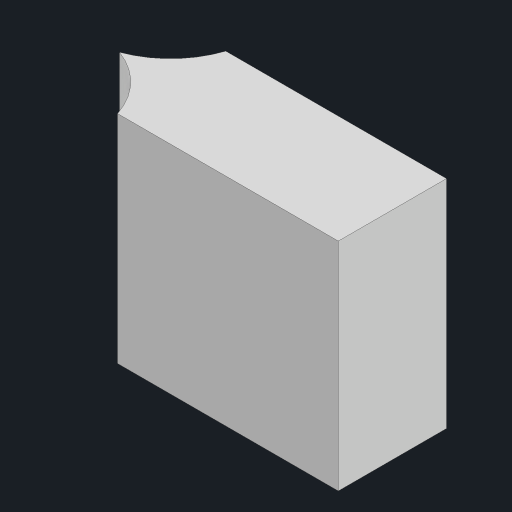
# Autodesk Inventor part: Capper Gate
Saved by Autodesk Inventor 2023.1 (Build 271208000, 208)
## iProperties
Created: 2023-02-21
Part Number: Capper Gate
Material: Generic
Document SubType Name: Modeling
Designer: Jarrett
Density: 1 g/cm^3
Appearance: Default
Author: Jarrett
Autodesk Inventor part; units mm, degrees
ref_plane "YZ Plane" through (0, 0, 0) normal (1, 0, 0) x (0, 1, 0)
ref_plane "XZ Plane" through (0, 0, 0) normal (0, 1, 0) x (-1, 0, 0)
ref_plane "XY Plane" through (0, 0, 0) normal (0, 0, 1) x (1, 0, 0)
sketch "Sketch2" plane through (0, 0, 0) normal (0, 1, 0) x (-1, 0, 0)
  circle A0 centre (0, -7.5) radius 7.5 construction
  line L0 (0, -19.5) -> (0, 12) projected
  arc A1 (-2.6473, 0.0493) -> (-7.5993, -5) centre (0, -7.5) ccw
  line L1 (-6.0208, -1.5) -> (-28, -1.5)
  line L2 (-6.0208, 0) -> (-6.0208, -1.5)
  line L3 (-6.0208, -1.5) -> (-5.6666, -1.8529) construction
  line L4 (14.6, 0) -> (-35.1, 0) projected
  line L5 (-28, -1.5) -> (-28, -5)
  line L6 (-28, -5) -> (-7.5993, -5)
  line L7 (-8, -7.5) -> (-8, -5) construction
  arc A2 (-7.5993, -5) -> (-8, -7.5) centre (0, -7.5) ccw construction
  line L8 (-8, -5.5) -> (-28, -5.5)
  line L9 (-28, -5.5) -> (-28, -7.5)
  line L10 (-28, -7.5) -> (-8, -7.5)
  line L11 (-14.0208, -1.5) -> (-14.0208, 0)
  line L12 (-10.0208, 0) -> (-10.0208, -1.5)
  line L13 (-28, -1.5) -> (-28, 0)
  arc A3 (-7.5993, 5) -> (-2.6473, -0.0493) centre (0, 7.5) ccw
  line L14 (-6.0208, 1.5) -> (-28, 1.5)
  line L15 (-6.0208, 0) -> (-6.0208, 1.5)
  line L16 (-28, 1.5) -> (-28, 5)
  line L17 (-28, 5) -> (-7.5993, 5)
  line L18 (-14.0208, 1.5) -> (-14.0208, 0)
  line L19 (-10.0208, 0) -> (-10.0208, 1.5)
  line L20 (-28, 1.5) -> (-28, 0)
  point P0 (0, 0)
  point P1 (-2.7839, 0)
  dimension "d0" = 15
  dimension "d2" = 0.5
  dimension "d4" = 0.5
  dimension "d5" = 3
  dimension "d6" = 10
  dimension "d8" = 20
  dimension "d9" = 0.5
  dimension "d11" = 8
  constraints: 38 end point, 9 vertical alignment, 8 point on circle, 7 point on line, 5 perpendicular, 4 vertical, 3 centre point, 2 horizontal, 2 line through centre, 1 collinear, 1 equal radius, 1 tangent, 8 other
  measures "d4" distance of L1.start L3.end
  measures "d8" distance of L9.end L7.start
  measures "d9" distance between parallel lines of L6 L8
  measures "d11" diameter of L2 L12
extrude "Extrusion1" add sketch "Sketch2" along normal blind 20
body "Solid1"
